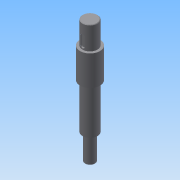
# Autodesk Inventor part: 齿轮160配件
Saved by Autodesk Inventor 2015 (Build 190159000, 159)
## iProperties
Created: 2017-05-27
Part Number: 齿轮160配件
Material: 常规
Document SubType Name: Modeling
Designer: Administrator
Density: 1 g/cm^3
Appearance: 默认
Author: Administrator
Autodesk Inventor part; units mm, degrees
ref_plane "YZ Plane" through (0, 0, 0) normal (1, 0, 0) x (0, 1, 0)
sketch "草图1" plane through (0, 0, 0) normal (0, 0, 1) x (1, 0, 0)
  circle A0 centre (0, 0) radius 10
  dimension "d0" = 20
  constraints: 1 centre point, 1 coincident
  measures "d0" diameter of A0
extrude "拉伸1" add sketch "草图1" along normal blind 51
sketch "草图2" plane through (0, 0, 51) normal (0, 0, 1) x (1, 0, 0)
  circle A0 centre (0, 0) radius 15
  dimension "d3" = 30
  constraints: 1 centre point, 1 coincident
  measures "d3" diameter of A0
extrude "拉伸2" add sketch "草图2" along normal blind 90
sketch "草图3" plane through (0, 0, 141) normal (0, 0, 1) x (1, 0, 0)
  circle A0 centre (0, 0) radius 20
  dimension "d6" = 40
  constraints: 1 centre point, 1 coincident
  measures "d6" diameter of A0
extrude "拉伸3" add sketch "草图3" along normal blind 60
sketch "草图4" plane through (0, 0, 201) normal (0, 0, 1) x (1, 0, 0)
  circle A0 centre (0, 0) radius 15
  dimension "d9" = 30
  constraints: 1 centre point, 1 coincident
  measures "d9" diameter of A0
extrude "拉伸4" add sketch "草图4" along normal blind 46
chamfer "倒角1" distance 1 angle 45 2 edges at (-15, 0, 247) (-10, 0, 0)
ref_plane "工作平面1" through (0, 10, 0) normal (0, 1, 0) x (-1, 0, 0)
sketch "草图5" plane through (0, 10, 0) normal (0, 1, 0) x (-1, 0, 0)
  line L0 (3, 44.5) -> (-3, 44.5)
  line L1 (-3, 44.5) -> (-3, 22.5)
  line L2 (-3, 22.5) -> (3, 22.5)
  line L3 (3, 22.5) -> (3, 44.5)
  arc A0 (-3, 22.5) -> (3, 22.5) centre (0, 22.5) ccw
  arc A1 (3, 44.5) -> (-3, 44.5) centre (0, 44.5) ccw
  line L4 (0, 0) -> (0, -6.1876)
  line L5 (-15, 51) -> (15, 51) projected
  dimension "d15" = 6
  dimension "d16" = 6.1876
  dimension "d17" = 6.5
  dimension "d18" = 22
  constraints: 10 end point, 4 point on circle, 4 tangent, 2 centre point, 2 parallel, 1 horizontal, 1 midpoint, 1 perpendicular, 1 point on line, 1 vertical
  measures "d15" distance of L0.start L0.end
  measures "d16" distance of L4.start L4.end
  measures "d17" distance from line of L5 A1.centre
  measures "d18" distance of L2.end L0.start
extrude "拉伸5" cut sketch "草图5" against normal blind 2.5
ref_plane "工作平面2" through (0, -15, 201) normal (0, 1, 0) x (-1, 0, 0)
sketch "草图6" plane through (0, -15, 201) normal (0, 1, 0) x (-1, 0, 0)
  line L0 (-4, 23.5) -> (4, 23.5)
  line L1 (4, 23.5) -> (4, 6.5)
  line L2 (4, 6.5) -> (-4, 6.5)
  line L3 (-4, 6.5) -> (-4, 23.5)
  arc A0 (-4, 6.5) -> (4, 6.5) centre (0, 6.5) ccw
  arc A1 (4, 23.5) -> (-4, 23.5) centre (0, 23.5) ccw
  line L4 (20, 0) -> (-20, 0) projected
  line L5 (0, 0) -> (0, 6.5)
  point P0 (0, -201)
  dimension "d21" = 6.5
  dimension "d22" = 8
  dimension "d23" = 17
  constraints: 10 end point, 4 point on circle, 4 tangent, 2 centre point, 2 midpoint, 2 parallel, 1 horizontal, 1 perpendicular, 1 vertical
  measures "d21" distance of L5.start L5.end
  measures "d22" distance of L1.end L2.end
  measures "d23" distance of L0.end L1.end
extrude "拉伸6" cut sketch "草图6" along normal blind 3
